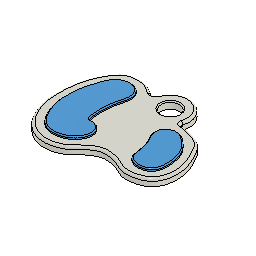
Mio Keychain v4 (Autodesk Fusion 360 design; units mm, degrees)
Autodesk Fusion 360 part; units mm, degrees
sketch "body" plane through (0, 0, 0) normal (0, 0, 1) x (1, 0, 0)
  arc A0 (3.080982, 4.614435) -> (-4.619204, 7.154245) centre (-0.795369, 5.804732) ccw
  arc A1 (-5.843525, 6.663859) -> (-4.619204, 7.154245) centre (-5.446522, 7.446223) ccw
  spline S0 degree 5 poles (-5.843525, 6.663859) (-5.915144, 6.710073) (-6.057081, 6.801322) (-6.266085, 6.934661) (-6.536953, 7.105373) (-6.8636, 7.306452) (-7.181547, 7.493641) (-7.497222, 7.663811) (-7.821491, 7.811675) (-8.166554, 7.931378) (-8.542705, 8.018119) (-8.954898, 8.069963) (-9.400086, 8.089017) (-9.870211, 8.078435) (-10.354714, 8.039623) (-10.843007, 7.969798) (-11.327499, 7.858377) (-11.804273, 7.687854) (-12.271353, 7.439199) (-12.727604, 7.096116) (-13.171414, 6.649581) (-13.599363, 6.102701) (-14.005237, 5.474142) (-14.381427, 4.792538) (-14.720048, 4.091957) (-15.014161, 3.406983) (-15.258963, 2.767917) (-15.452961, 2.196022) (-15.599228, 1.698524) (-15.706419, 1.264339) (-15.786087, 0.871329) (-15.850057, 0.493271) (-15.908051, 0.106313) (-15.964539, -0.302854) (-16.018798, -0.735962) (-16.067511, -1.187719) (-16.106576, -1.64871) (-16.133361, -2.109069) (-16.148444, -2.561543) (-16.15412, -3.001519) (-16.153102, -3.427316) (-16.14727, -3.840283) (-16.136088, -4.245219) (-16.116572, -4.649581) (-16.084416, -5.061794) (-16.034741, -5.489896) (-15.963095, -5.939879) (-15.866028, -6.414689) (-15.74095, -6.914512) (-15.586116, -7.436779) (-15.400569, -7.976316) (-15.184097, -8.525364) (-14.937188, -9.073845) (-14.66103, -9.610632) (-14.35749, -10.124659) (-14.029121, -10.606143) (-13.679124, -11.047659) (-13.311399, -11.4455) (-12.930343, -11.800212) (-12.540013, -12.114927) (-12.143382, -12.394103) (-11.741603, -12.642135) (-11.333163, -12.861935) (-10.913403, -13.053784) (-10.476269, -13.21605) (-10.015868, -13.345701) (-9.527988, -13.438886) (-9.011891, -13.491498) (-8.471124, -13.499733) (-7.912511, -13.460649) (-7.345539, -13.372712) (-6.78161, -13.236375) (-6.233299, -13.054583) (-5.713738, -12.833471) (-5.234854, -12.581386) (-4.805495, -12.30765) (-4.429429, -12.021354) (-4.103783, -11.730274) (-3.816318, -11.439398) (-3.547615, -11.151129) (-3.277025, -10.866695) (-2.986999, -10.587145) (-2.669254, -10.314671) (-2.326038, -10.053224) (-1.964227, -9.808184) (-1.591155, -9.586238) (-1.209648, -9.395195) (-0.813668, -9.243771) (-0.393525, -9.139829) (0.058742, -9.088514) (0.544791, -9.090723) (1.053263, -9.140708) (1.561734, -9.227194) (2.044846, -9.336963) (2.481012, -9.457938) (2.858864, -9.581997) (3.185949, -9.709094) (3.485309, -9.844637) (3.785957, -9.993503) (4.115353, -10.155165) (4.490888, -10.318223) (4.920977, -10.464877) (5.406167, -10.575724) (5.940287, -10.634024) (6.511463, -10.631197) (7.103633, -10.567992) (7.698672, -10.450497) (8.278319, -10.287542) (8.826284, -10.087394) (9.330044, -9.855095) (9.783372, -9.588662) (10.185581, -9.280039) (10.539063, -8.918512) (10.847267, -8.49347) (11.112684, -7.997203) (11.334364, -7.428242) (11.507326, -6.792456) (11.624716, -6.100845) (11.679316, -5.368134) (11.665266, -4.611069) (11.579812, -3.84679) (11.42477, -3.091288) (11.208788, -2.357533) (10.946471, -1.654973) (10.65485, -0.990218) (10.350562, -0.367391) (10.046842, 0.211393) (9.750342, 0.745597) (9.458619, 1.235817) (9.155841, 1.683325) (8.816018, 2.089713) (8.411418, 2.45659) (7.919343, 2.785275) (7.329804, 3.076481) (6.652285, 3.330033) (5.924337, 3.544473) (5.20057, 3.71803) (4.53898, 3.849799) (4.053497, 3.930072) (3.75835, 3.970794) (3.588366, 3.990779) (3.500024, 4.000038) (3.475103, 4.002551) knots 0 0 0 0 0 0 0.00714286 0.01428571 0.02142857 0.02857143 0.03571429 0.04285714 0.05 0.05714286 0.06428571 0.07142857 0.07857143 0.08571429 0.09285714 0.1 0.10714286 0.11428571 0.12142857 0.12857143 0.13571429 0.14285714 0.15 0.15714286 0.16428571 0.17142857 0.17857143 0.18571429 0.19285714 0.2 0.20714286 0.21428571 0.22142857 0.22857143 0.23571429 0.24285714 0.25 0.25714286 0.26428571 0.27142857 0.27857143 0.28571429 0.29285714 0.3 0.30714286 0.31428571 0.32142857 0.32857143 0.33571429 0.34285714 0.35 0.35714286 0.36428571 0.37142857 0.37857143 0.38571429 0.39285714 0.4 0.40714286 0.41428571 0.42142857 0.42857143 0.43571429 0.44285714 0.45 0.45714286 0.46428571 0.47142857 0.47857143 0.48571429 0.49285714 0.5 0.50714286 0.51428571 0.52142857 0.52857143 0.53571429 0.54285714 0.55 0.55714286 0.56428571 0.57142857 0.57857143 0.58571429 0.59285714 0.6 0.60714286 0.61428571 0.62142857 0.62857143 0.63571429 0.64285714 0.65 0.65714286 0.66428571 0.67142857 0.67857143 0.68571429 0.69285714 0.7 0.70714286 0.71428571 0.72142857 0.72857143 0.73571429 0.74285714 0.75 0.75714286 0.76428571 0.77142857 0.77857143 0.78571429 0.79285714 0.8 0.80714286 0.81428571 0.82142857 0.82857143 0.83571429 0.84285714 0.85 0.85714286 0.86428571 0.87142857 0.87857143 0.88571429 0.89285714 0.9 0.90714286 0.91428571 0.92142857 0.92857143 0.93571429 0.94285714 0.95 0.95714286 0.96428571 0.97142857 0.97857143 0.98152044 0.98152044 0.98152044 0.98152044 0.98152044 0.98152044
  circle A2 centre (-0.795369, 5.804732) radius 1.967471
  arc A3 (3.080982, 4.614435) -> (3.5, 4) centre (3.536072, 4.474693) ccw
extrude "Extrude1" add sketch "body" along normal blind 1.5
sketch "i left" plane through (0, 0, 1.5) normal (0, 0, 1) x (1, 0, 0)
  spline S0 degree 5 poles (-13.8, 0.01) (-13.813154, -0.04565) (-13.837565, -0.152725) (-13.86877, -0.302511) (-13.901473, -0.491005) (-13.933995, -0.739787) (-13.964357, -1.030932) (-13.996005, -1.3803) (-14.028896, -1.787658) (-14.060674, -2.242831) (-14.087354, -2.729531) (-14.104201, -3.230084) (-14.106532, -3.729874) (-14.090516, -4.221617) (-14.053097, -4.70347) (-13.991977, -5.177486) (-13.905568, -5.647942) (-13.792968, -6.119718) (-13.653912, -6.596666) (-13.488754, -7.079933) (-13.298196, -7.568227) (-13.083008, -8.058162) (-12.843768, -8.544582) (-12.580564, -9.020883) (-12.292767, -9.479349) (-11.978651, -9.911455) (-11.635493, -10.308269) (-11.260444, -10.661036) (-10.851223, -10.961711) (-10.406887, -11.203513) (-9.928559, -11.381473) (-9.420193, -11.492995) (-8.889278, -11.538373) (-8.3458, -11.520121) (-7.801256, -11.44233) (-7.267669, -11.310029) (-6.75656, -11.128518) (-6.278031, -10.902777) (-5.839572, -10.636675) (-5.445847, -10.332917) (-5.099681, -9.993908) (-4.802716, -9.622365) (-4.556249, -9.222071) (-4.361888, -8.798475) (-4.222537, -8.359589) (-4.142311, -7.915936) (-4.125049, -7.479281) (-4.173174, -7.061668) (-4.286421, -6.674335) (-4.460591, -6.326663) (-4.686383, -6.025165) (-4.950856, -5.77382) (-5.238773, -5.57439) (-5.534005, -5.426666) (-5.820862, -5.328908) (-6.085659, -5.277607) (-6.318721, -5.266368) (-6.51606, -5.285092) (-6.681721, -5.318883) (-6.824156, -5.346859) (-6.950966, -5.339191) (-7.065757, -5.259278) (-7.169848, -5.082646) (-7.263069, -4.810084) (-7.344329, -4.458001) (-7.412094, -4.050725) (-7.46492, -3.611671) (-7.5019, -3.156205) (-7.522646, -2.694141) (-7.527308, -2.231232) (-7.516585, -1.771122) (-7.491721, -1.316915) (-7.454564, -0.873356) (-7.407412, -0.447189) (-7.352575, -0.044875) (-7.291972, 0.329138) (-7.226775, 0.674218) (-7.156893, 0.995685) (-7.080952, 1.30571) (-6.998271, 1.619103) (-6.910604, 1.949781) (-6.823836, 2.307143) (-6.750077, 2.692018) (-6.705126, 3.09825) (-6.70534, 3.515047) (-6.764616, 3.929088) (-6.891561, 4.326651) (-7.085968, 4.695954) (-7.340561, 5.027482) (-7.643817, 5.313847) (-7.982507, 5.549831) (-8.344136, 5.732312) (-8.719987, 5.860346) (-9.1049, 5.934649) (-9.495625, 5.95686) (-9.889562, 5.928839) (-10.283483, 5.852016) (-10.671914, 5.726545) (-11.04769, 5.551631) (-11.40332, 5.326306) (-11.732135, 5.050073) (-12.029405, 4.723564) (-12.293783, 4.349296) (-12.527345, 3.932001) (-12.734186, 3.478565) (-12.91943, 2.998041) (-13.08803, 2.501697) (-13.24376, 2.002908) (-13.387867, 1.51746) (-13.518762, 1.062486) (-13.633613, 0.652838) (-13.710341, 0.368992) (-13.758637, 0.181176) (-13.786845, 0.06565) (-13.8, 0.01) knots 0 0 0 0 0 0 0.00909091 0.01818182 0.02727273 0.03636364 0.04545455 0.05454545 0.06363636 0.07272727 0.08181818 0.09090909 0.1 0.10909091 0.11818182 0.12727273 0.13636364 0.14545455 0.15454545 0.16363636 0.17272727 0.18181818 0.19090909 0.2 0.20909091 0.21818182 0.22727273 0.23636364 0.24545455 0.25454545 0.26363636 0.27272727 0.28181818 0.29090909 0.3 0.30909091 0.31818182 0.32727273 0.33636364 0.34545455 0.35454545 0.36363636 0.37272727 0.38181818 0.39090909 0.4 0.40909091 0.41818182 0.42727273 0.43636364 0.44545455 0.45454545 0.46363636 0.47272727 0.48181818 0.49090909 0.5 0.50909091 0.51818182 0.52727273 0.53636364 0.54545455 0.55454545 0.56363636 0.57272727 0.58181818 0.59090909 0.6 0.60909091 0.61818182 0.62727273 0.63636364 0.64545455 0.65454545 0.66363636 0.67272727 0.68181818 0.69090909 0.7 0.70909091 0.71818182 0.72727273 0.73636364 0.74545455 0.75454545 0.76363636 0.77272727 0.78181818 0.79090909 0.8 0.80909091 0.81818182 0.82727273 0.83636364 0.84545455 0.85454545 0.86363636 0.87272727 0.88181818 0.89090909 0.9 0.90909091 0.91818182 0.92727273 0.93636364 0.94545455 0.95454545 0.96363636 0.97272727 0.98181818 0.99090909 1 1 1 1 1 1
extrude "Extrude2" add sketch "i left" along normal blind 0.5
sketch "i right" plane through (0, 0, 1.5) normal (0, 0, 1) x (1, 0, 0)
  spline S0 degree 5 poles (2.983649, -2.730149) (3.010873, -2.780183) (3.06527, -2.882478) (3.146425, -3.043592) (3.252513, -3.276287) (3.378336, -3.597441) (3.494361, -3.944924) (3.598209, -4.31172) (3.6885, -4.689084) (3.765304, -5.06803) (3.83024, -5.440226) (3.886217, -5.798344) (3.937268, -6.136531) (3.988361, -6.450871) (4.045195, -6.739777) (4.114053, -7.004601) (4.201292, -7.248608) (4.312752, -7.475553) (4.453226, -7.688508) (4.625808, -7.888315) (4.831654, -8.073136) (5.070372, -8.239548) (5.340263, -8.383294) (5.638606, -8.50013) (5.96196, -8.586735) (6.306138, -8.640671) (6.666104, -8.660112) (7.03588, -8.643649) (7.408484, -8.59009) (7.775772, -8.4982) (8.128586, -8.366654) (8.457701, -8.194566) (8.754605, -7.981889) (9.012387, -7.729898) (9.226482, -7.441567) (9.395719, -7.122173) (9.522192, -6.779028) (9.610206, -6.420548) (9.66551, -6.055517) (9.694397, -5.692264) (9.702894, -5.337903) (9.695827, -4.997471) (9.676867, -4.673908) (9.648705, -4.368175) (9.613202, -4.079295) (9.571516, -3.804473) (9.524301, -3.539067) (9.471561, -3.277285) (9.412362, -3.01319) (9.34462, -2.74157) (9.264781, -2.45895) (9.167768, -2.164293) (9.048064, -1.858423) (8.90064, -1.54363) (8.721953, -1.223197) (8.510877, -0.900972) (8.269767, -0.580904) (8.003575, -0.266948) (7.718825, 0.037005) (7.422665, 0.327202) (7.121841, 0.600108) (6.821805, 0.852472) (6.525511, 1.081422) (6.23351, 1.284468) (5.944926, 1.459448) (5.658165, 1.60449) (5.371731, 1.717979) (5.085019, 1.798498) (4.799035, 1.84483) (4.516065, 1.856348) (4.239458, 1.83341) (3.973324, 1.777691) (3.722363, 1.692699) (3.491237, 1.583611) (3.283302, 1.456343) (3.099654, 1.316814) (2.937704, 1.170137) (2.79108, 1.019809) (2.653401, 0.866446) (2.520918, 0.706955) (2.396554, 0.532752) (2.289055, 0.331903) (2.208766, 0.094275) (2.164692, -0.18476) (2.160317, -0.498713) (2.193792, -0.832149) (2.259909, -1.166086) (2.351559, -1.482607) (2.461281, -1.769268) (2.58308, -2.024911) (2.71277, -2.25908) (2.820305, -2.441203) (2.901925, -2.582275) (2.956425, -2.680116) (2.983649, -2.730149) knots 0 0 0 0 0 0 0.01111111 0.02222222 0.03333333 0.04444444 0.05555556 0.06666667 0.07777778 0.08888889 0.1 0.11111111 0.12222222 0.13333333 0.14444444 0.15555556 0.16666667 0.17777778 0.18888889 0.2 0.21111111 0.22222222 0.23333333 0.24444444 0.25555556 0.26666667 0.27777778 0.28888889 0.3 0.31111111 0.32222222 0.33333333 0.34444444 0.35555556 0.36666667 0.37777778 0.38888889 0.4 0.41111111 0.42222222 0.43333333 0.44444444 0.45555556 0.46666667 0.47777778 0.48888889 0.5 0.51111111 0.52222222 0.53333333 0.54444444 0.55555556 0.56666667 0.57777778 0.58888889 0.6 0.61111111 0.62222222 0.63333333 0.64444444 0.65555556 0.66666667 0.67777778 0.68888889 0.7 0.71111111 0.72222222 0.73333333 0.74444444 0.75555556 0.76666667 0.77777778 0.78888889 0.8 0.81111111 0.82222222 0.83333333 0.84444444 0.85555556 0.86666667 0.87777778 0.88888889 0.9 0.91111111 0.92222222 0.93333333 0.94444444 0.95555556 0.96666667 0.97777778 0.98888889 1 1 1 1 1 1
extrude "Extrude3" add sketch "i right" along normal blind 0.5
fillet "Fillet1" radius 0.5 4 edges at (-6.971833, -13.27554, 1.5) (3.142762, 4.206473, 1.5) (0.474808, 9.655648, 1.5) (-5.120313, 6.631796, 1.5)
fillet "Fillet2" radius 0.22 1 edges at (-2.629696, 6.5162, 1.5)
fillet "Fillet3" radius 0.22 1 edges at (-6.508177, -5.288809, 2)
fillet "Fillet4" radius 0.22 1 edges at (9.469936, -3.276713, 2)
